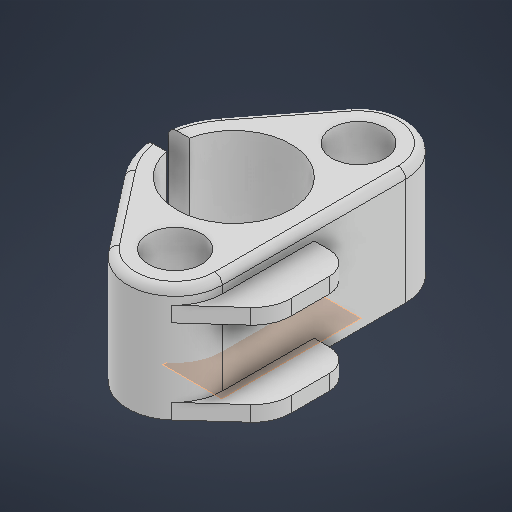
# Autodesk Inventor part: PresaPilotInventorVersion
Saved by Autodesk Inventor 2026.2 (Build 302298000, 298)
## iProperties
Created: 2026-04-15
Part Number: PresaPilotInventorVersion
Material: Generic
Document SubType Name: Modeling
Designer: 06aar
Density: 1 g/cm^3
Appearance: Default
Author: 06aar
Autodesk Inventor part; units mm, degrees
ref_plane "YZ Plane" through (0, 0, 0) normal (1, 0, 0) x (0, 1, 0)
ref_plane "XZ Plane" through (0, 0, 0) normal (0, 1, 0) x (-1, 0, 0)
ref_plane "XY Plane" through (0, 0, 0) normal (0, 0, 1) x (1, 0, 0)
sketch "Sketch1" plane through (0, 0, 0) normal (0, 1, 0) x (-1, 0, 0)
  circle A0 centre (0, 0) radius 7.45
  line L0 (0, 0) -> (-4.32, 12)
  circle A1 centre (-4.32, 12) radius 3.48
  circle A2 centre (-4.32, 12) radius 6.18
  line L1 (-10.5, 28.575) -> (-10.5, -28.575)
  line L2 (7.45, 0) -> (-7.45, 0)
  circle A3 centre (0, 0) radius 10.15
  line L3 (0.5542, 15.7993) -> (8.0054, 6.2399)
  circle A4 centre (-4.32, -12) radius 3.48
  circle A5 centre (-4.32, -12) radius 6.18
  line L4 (0.5542, -15.7993) -> (8.0054, -6.2399)
  point P0 (-10.5, 0)
  point P1 (-10.5, 12)
  point P2 (-10.5, -12)
  dimension "d0" = 14.9
  dimension "d7" = 2.7
  dimension "d1" = 6.96
  dimension "d3" = 10.5
  dimension "d5" = 2.7
  dimension "d6" = 12
  constraints: 10 end point, 5 coincident, 4 symmetric about line, 2 centre point, 2 horizontal, 2 midpoint, 2 vertical, 1 horizontal alignment, 14 other
  measures "d1" diameter of A1
  measures "d3" distance from line of L1 point (0, 0)
  measures "d6" distance from line of L2 L0.end
extrude "Extrusion1" add sketch "Sketch1" along normal blind 15 contours A0 A2 A3 A5 | A0 L0 A1 A3 A2 | A5 A3 A4 A0 | A0 A2 A3 A1 L0 | A3 A1 A2 | A2 L3 A3 | A5 A3 A2 A0 | A5 A3 A4 | A3 L4 A5 | A5 L1 A2 A3
sketch "Sketch2" plane through (0, 0, 0) normal (0, -1, 0) x (1, 0, 0)
  arc A0 (10.5, 12) -> (-0.5542, 15.7993) centre (4.32, 12) ccw projected
  line L0 (8.4662, 16.5827) -> (13.8545, 11.7077)
  line L1 (15.5, 8) -> (15.5, 3)
  line L2 (10.5, 12) -> (10.5, -12) projected
  arc A1 (15.5, 8) -> (13.8545, 11.7077) centre (10.5, 8) ccw
  line L3 (10.5, 0) -> (12.5, 0)
  arc A2 (12.5, 0) -> (15.5, 3) centre (12.5, 3) ccw
  line L4 (10.5, -12) -> (10.5, 12)
  arc A3 (10.5, 12) -> (-0.5542, 15.7993) centre (4.32, 12) ccw
  point P0 (0, 0)
  point P1 (15.5, 0)
  dimension "d10" = 5
  dimension "d11" = 5
  dimension "d12" = 8
  dimension "d13" = 3
  dimension "d14" = 0
  constraints: 8 end point, 7 point on circle, 5 tangent, 3 centre point, 2 point on line, 1 horizontal, 1 midpoint, 1 vertical, 1 other
  measures "d10" distance between parallel lines of L2 L1
  measures "d11" radius of A1
  measures "d12" distance of L1.start point (15.5, 0)
  measures "d13" radius of A2
  measures "d14" radial gap between concentric circles of A0 A3
extrude "Extrusion2" add sketch "Sketch2" against normal blind 2
ref_plane "Work Plane1" through (0, 6.5, 0) normal (0, 1, 0) x (1, 0, 0)
mirror "Mirror1" about plane through (0, 6.5, 0) normal (0, 1, 0) of "Extrusion2"
fillet "Fillet1" radius 1 6 edges at (6.3287, 15, -17.8444) (-4.2798, 15, -11.0196) (-10.15, 15, 0) (-4.2798, 15, 11.0196) (6.3287, 15, 17.8444) (10.5, 15, 0)
sketch "Sketch3" plane through (0, 15, 0) normal (0, 1, 0) x (1, 0, 0)
  line L0 (-17.025, 1.5) -> (-2.025, 1.5)
  line L1 (-2.025, 1.5) -> (-2.025, -1.5)
  line L2 (-2.025, -1.5) -> (-17.025, -1.5)
  line L3 (-17.025, -1.5) -> (-17.025, 1.5)
  line L4 (-17.025, 1.5) -> (-2.025, -1.5) construction
  line L5 (-2.025, 1.5) -> (-17.025, -1.5) construction
  point P0 (0, 0)
  point P1 (-9.525, 0)
  dimension "d19" = 3
  dimension "d20" = 1.5
  dimension "d21" = 15
  constraints: 12 end point, 2 midpoint, 2 parallel, 1 horizontal, 1 perpendicular
  measures "d19" distance between parallel lines of L2 L0
  measures "d20" distance from line of L0 point (-9.525, 0)
  measures "d21" distance of L0.start L0.end
extrude "Extrusion3" cut sketch "Sketch3" against normal through all
body "Solid1"
